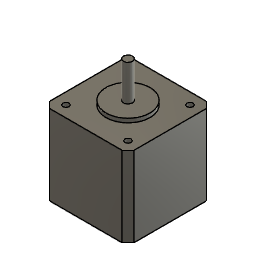
nema17stepper v1 (Autodesk Fusion 360 design; units mm, degrees)
Autodesk Fusion 360 part; units mm, degrees
sketch "スケッチ1" plane through (0, 0, 0) normal (0, 1, 0) x (1, 0, 0)
  line L0 (0, 0) -> (21.15, 0)
  line L1 (21.15, 0) -> (21.15, 21.15)
  line L2 (21.15, 21.15) -> (0, 21.15)
  line L3 (0, 21.15) -> (0, 0)
  line L4 (0, 0) -> (15.5, 0) construction
  line L5 (15.5, 0) -> (15.5, 15.5) construction
  line L6 (15.5, 15.5) -> (0, 15.5) construction
  line L7 (0, 15.5) -> (0, 0) construction
  circle A0 centre (15.5, 15.5) radius 1.5
  dimension "d1" = 21.15
  dimension "d2" = 21.15
  dimension "d3" = 15.5
  dimension "d4" = 15.5
  dimension "d5" = 3
  constraint horizontal L0
  constraint vertical L1
  constraint horizontal L2
  constraint vertical L3
  constraint coincident L0.start L3.end
  constraint horizontal L4
  constraint vertical L5
  constraint horizontal L6
  constraint vertical L7
  constraint coincident L5.end L6.start
  measures "d1" distance of L0.start L0.end
  measures "d2" distance of L0.start L2.end
  measures "d3" distance of L0.start L4.end
  measures "d4" distance of L0.start L6.end
  measures "d5" diameter of A0
extrude "押し出し1" add sketch "スケッチ1" along normal blind 40 contours L0 L1 L2 L3 | A0 makes body 1
mirror "ミラー1" about plane through (0, 0, 0) normal (0, 0, -1) of bodies 1 makes body 2
mirror "ミラー2" about plane through (0, 0, 21.15) normal (-1, 0, 0) of bodies 1 2 makes body 3 at (0, 13.3333, -14.1) makes body 4 at (0, 13.3333, 14.1)
combine "結合1" operation add target body 4 tool bodies 1 2 3
sketch "スケッチ2" plane through (0, 40, 0) normal (0, 1, 0) x (-1, 0, 0)
  line L0 (-21.15, -21.15) -> (21.15, -21.15)
  line L1 (21.15, -21.15) -> (21.15, 21.15)
  line L2 (21.15, 21.15) -> (-21.15, 21.15)
  line L3 (-21.15, 21.15) -> (-21.15, -21.15)
  circle A0 centre (0, 0) radius 11
  line L4 (15.5, 15.5) -> (-15.5, 15.5) construction
  line L5 (-15.5, 15.5) -> (-15.5, -15.5) construction
  line L6 (-15.5, -15.5) -> (15.5, -15.5) construction
  line L7 (15.5, -15.5) -> (15.5, 15.5) construction
  line L8 (15.5, 15.5) -> (-15.5, -15.5) construction
  line L9 (-15.5, 15.5) -> (15.5, -15.5) construction
  circle A1 centre (15.5, -15.5) radius 1.5
  circle A2 centre (-15.5, -15.5) radius 1.5
  circle A3 centre (15.5, 15.5) radius 1.5
  circle A4 centre (-15.5, 15.5) radius 1.5
  circle A5 centre (0, 0) radius 2.25
  dimension "d10" = 22
  dimension "d13" = 31
  dimension "d14" = 31
  dimension "d15" = 3
  dimension "d16" = 3
  dimension "d17" = 3
  dimension "d18" = 3
  dimension "d21" = 4.5
  constraint coincident A0.centre A5.centre
  constraint horizontal L4
  constraint perpendicular L4 L5
  constraint parallel L4 L6
  constraint parallel L5 L7
  constraint coincident L8 A0.centre
  constraint coincident L9 A0.centre
  constraint coincident L6.end L7.start
  constraint coincident L5.end L6.start
  constraint coincident L4.start L7.end
  constraint coincident L4.end L5.start
  measures "d10" diameter of A0
  measures "d13" distance of L5.end L6.end
  measures "d14" distance of L4.end L5.end
  measures "d15" diameter of A1
  measures "d16" diameter of A2
  measures "d17" diameter of A3
  measures "d18" diameter of A4
  measures "d21" diameter of A5
extrude "押し出し2" add sketch "スケッチ2" along normal blind 2 contours A0 | A5 bodies 4
extrude "押し出し3" cut sketch "スケッチ2" against normal blind 4.5 contours A1 | A2 | A3 | A4 bodies 4
extrude "押し出し4" add sketch "スケッチ2" along normal blind 20 contours A5 bodies 4
chamfer "面取り1" distance 3 angle 45 4 edges at (-21.15, 20, -21.15) (-21.15, 20, 21.15) (21.15, 20, 21.15) (21.15, 20, -21.15) on bodies 4
equation "d1 = ( 42.3 / 2 ) * 1 mm"
equation "d2 = ( 42.3 / 2 ) * 1 mm"
equation "d3 = ( 31 / 2 ) * 1 mm"
equation "d4 = ( 31 / 2 ) * 1 mm"
